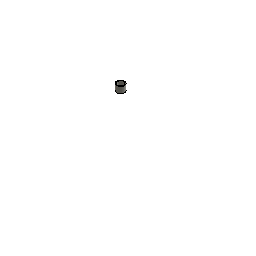
Axis2tube (Autodesk Fusion 360 design; units mm, degrees)
Autodesk Fusion 360 part; units mm, degrees
sketch "Sketch1" plane through (0, 0, 110) normal (0, -1, 0) x (1, 0, 0)
  circle A0 centre (0, -110) radius 5
  circle A1 centre (0, -110) radius 13
  circle A2 centre (0, -110) radius 4
  circle A3 centre (0, -110) radius 5
  dimension "d1029" = 1
  dimension "d1030" = 10
  measures "d1029" distance of A2 A3
  measures "d1030" diameter of A3
extrude "Extrude1" add sketch "Sketch1" against normal up to surface (8 mm away) contours A0 A3
chamfer "Chamfer1" distance 0.5 angle 45 1 edges at (-3.7293, 0, 1.4465)
sketch "Sketch2" plane through (0, -121, 0) normal (0, -1, 0) x (1, 0, 0)
  circle A0 centre (0, -25) radius 1.575
  circle A1 centre (0, -25) radius 3.75
  circle A2 centre (0, -25) radius 1.575
extrude "Extrude2" cut sketch "Sketch2" along normal up to surface contours A0 A2 end surface at (3.9801, 5.5, -0.3983)
sketch "Sketch3" plane through (0, -96.5, 0) normal (0, 1, 0) x (-1, 0, 0)
  line L0 (12.8475, 19.9) -> (12.8475, 16.9)
  line L1 (12.8475, 16.9) -> (6.2657, 16.9)
  line L2 (6.2657, 16.9) -> (6.2657, 19.9)
  line L3 (6.2657, 19.9) -> (12.8475, 19.9)
  line L4 (-6.2657, 19.9) -> (-6.2657, 16.9)
  line L5 (-6.2657, 16.9) -> (-12.8475, 16.9)
  line L6 (-12.8475, 16.9) -> (-12.8475, 19.9)
  line L7 (-12.8475, 19.9) -> (-6.2657, 19.9)
  line L8 (-6.2657, -26.9) -> (-6.2657, -29.9)
  line L9 (-6.2657, -29.9) -> (-12.8475, -29.9)
  line L10 (-12.8475, -29.9) -> (-12.8475, -26.9)
  line L11 (-12.8475, -26.9) -> (-6.2657, -26.9)
  line L12 (6.2657, -29.9) -> (6.2657, -26.9)
  line L13 (6.2657, -26.9) -> (12.8475, -26.9)
  line L14 (12.8475, -26.9) -> (12.8475, -29.9)
  line L15 (12.8475, -29.9) -> (6.2657, -29.9)
  line L16 (-5.15, -39.9) -> (-5.15, -10)
  arc A0 (5.15, -10) -> (-5.15, -10) centre (0, -10) ccw
  line L17 (5.15, -10) -> (5.15, -39.9)
  line L18 (5.15, -39.9) -> (21, -39.9)
  line L19 (21, -39.9) -> (21, 29.9)
  line L20 (21, 29.9) -> (-22.2672, 29.9)
  line L21 (-22.2672, 29.9) -> (-22.2672, -39.9)
  line L22 (-22.2672, -39.9) -> (-5.15, -39.9)
  circle A1 centre (0, -10) radius 4
  dimension "d1036" = 8
  measures "d1036" diameter of A1
extrude "Extrude3" cut sketch "Sketch3" along normal up to surface contours A1 end surface at (3.9801, 5.5, -0.3983)
